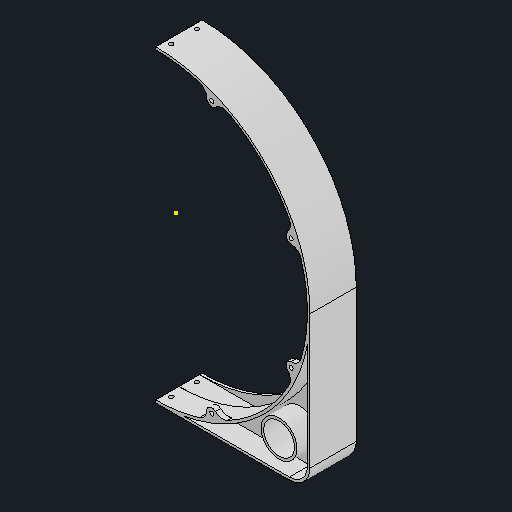
# Autodesk Inventor part: 3DPRINT,CABLE-SHROUD,OUTER
Saved by Autodesk Inventor 2026 (Build 300175000, 175)
## iProperties
Created: 2026-02-11
Part Number: 3DPRINT,CABLE-SHROUD,OUTER
Material: Generic
Document SubType Name: Modeling
Designer: littl
Density: 1 g/cm^3
Appearance: Default
Mass: 377.727 g
Surface Area: 2418.76 cm^2
Volume: 377.727 cm^3
Author: littl
Autodesk Inventor part; units mm, degrees
ref_plane "YZ Plane" through (0, 0, 0) normal (1, 0, 0) x (0, 1, 0)
ref_plane "XZ Plane" through (0, 0, 0) normal (0, 1, 0) x (-1, 0, 0)
ref_plane "XY Plane" through (0, 0, 0) normal (0, 0, 1) x (1, 0, 0)
sketch "Sketch1" plane through (0, 0, 0) normal (0, 0, 1) x (1, 0, 0)
  arc A0 (190.5, 0) -> (-190.5, 0) centre (0, 0) ccw
  circle A1 centre (0, 0) radius 187.325
  line L0 (-190.5, 0) -> (-190.5, -165.1)
  line L1 (-165.1, -190.5) -> (165.1, -190.5)
  line L2 (190.5, -165.1) -> (190.5, 0)
  arc A2 (-190.5, -165.1) -> (-165.1, -190.5) centre (-165.1, -165.1) ccw
  arc A3 (165.1, -190.5) -> (190.5, -165.1) centre (165.1, -165.1) ccw
  dimension "d0" = 381
  dimension "d1" = 3.175
  dimension "d2" = 25.4
  constraints: 7 tangent, 6 end point, 6 point on circle, 4 centre point, 2 coincident, 2 perpendicular, 1 equal radius, 1 vertical
  measures "d0" diameter of A0
  measures "d1" radial gap between concentric circles of A1 A0
  measures "d2" radius of A2
extrude "Extrusion1" add sketch "Sketch1" along normal blind 3.175
sketch "Sketch2" plane through (0, 0, 3.175) normal (0, 0, 1) x (1, 0, 0)
  line L0 (-190.5, 0) -> (-190.5, -165.1) projected
  arc A0 (-190.5, -165.1) -> (-165.1, -190.5) centre (-165.1, -165.1) ccw projected
  line L1 (-165.1, -190.5) -> (165.1, -190.5) projected
  arc A1 (165.1, -190.5) -> (190.5, -165.1) centre (165.1, -165.1) ccw projected
  line L2 (190.5, -165.1) -> (190.5, 0) projected
  arc A2 (190.5, 0) -> (-190.5, 0) centre (0, 0) ccw projected
  circle A3 centre (0, 0) radius 187.325 projected
  line L3 (-187.325, 0) -> (-187.325, -161.925)
  line L4 (187.325, 0) -> (187.325, -161.925)
  line L5 (161.925, -187.325) -> (-161.925, -187.325)
  circle A4 centre (0, 0) radius 187.325 projected
  arc A5 (-187.325, -161.925) -> (-161.925, -187.325) centre (-161.925, -161.925) ccw
  arc A6 (161.925, -187.325) -> (187.325, -161.925) centre (161.925, -161.925) ccw
  dimension "d5" = 25.4
  constraints: 7 tangent, 6 end point, 6 point on circle, 2 centre point, 2 perpendicular, 1 equal radius, 1 vertical
  measures "d5" radius of A5
extrude "Extrusion2" add sketch "Sketch2" along normal blind 12.7
mirror "Mirror1" about plane through (0, 0, 15.875) normal (0, 0, 1) of "Extrusion1", "Extrusion2"
sketch "Sketch3" plane through (0, 0, 31.75) normal (0, 0, 1) x (1, 0, 0)
  point P0 (0, 0)
sketch "Sketch4" plane through (0, 0, 31.75) normal (0, 0, -1) x (-1, 0, 0)
  line L0 (190.5, 0) -> (190.5, -165.1) projected
  arc A0 (190.5, 0) -> (-190.5, 0) centre (0, 0) ccw projected
  line L1 (-190.5, -165.1) -> (-190.5, 0) projected
  arc A1 (-190.5, -165.1) -> (-165.1, -190.5) centre (-165.1, -165.1) ccw projected
  line L2 (165.1, -190.5) -> (-165.1, -190.5) projected
  arc A2 (165.1, -190.5) -> (190.5, -165.1) centre (165.1, -165.1) ccw projected
  circle A3 centre (0, 0) radius 187.325 projected
  arc A4 (-187.325, -165.1) -> (-165.1, -187.325) centre (-165.1, -165.1) ccw
  line L3 (-187.325, -165.1) -> (-187.325, 0)
  arc A5 (187.325, 0) -> (-187.325, 0) centre (0, 0) ccw
  line L4 (187.325, 0) -> (187.325, -165.1)
  arc A6 (165.1, -187.325) -> (187.325, -165.1) centre (165.1, -165.1) ccw
  line L5 (165.1, -187.325) -> (-165.1, -187.325)
  circle A7 centre (0, 0) radius 190.5
  point P0 (-34.6352, -187.325)
  point P1 (-187.325, -34.6352)
  point P2 (34.6352, -187.325)
  point P3 (187.325, -34.6352)
  dimension "d8" = 3.175
  dimension "d9" = 3.175
  constraints: 6 end point, 6 point on circle, 4 centre point, 5 other
  measures "d8" distance between parallel lines of L2 L5
  measures "d9" radial gap between concentric circles of A3 A7
extrude "Extrusion3" add sketch "Sketch4" against normal blind 25.4504 contours A7 L4 A3 L3 A0 | L0 A2 L2 A7 L5 A6 L4 | A7 L3 A4 L5 L2 A1 L1 | A7 L5 A3 L4 | L3 A3 L5 A7 | A7 L5
sketch "Sketch5" plane through (161.925, -187.325, 28.575) normal (0, 0, -1) x (-1, 0, 0)
  circle A0 centre (9.525, 34.925) radius 19.05
  point P0 (161.925, 187.325)
  dimension "d12" = 38.1
  dimension "d13" = 152.4
  dimension "d14" = 152.4
  constraints: 1 centre point
  measures "d12" diameter of A0
  measures "d13" horizontal distance of point (161.925, 187.325) A0.centre
  measures "d14" horizontal distance of point (161.925, 187.325) A0.centre
extrude "Extrusion4" cut sketch "Sketch5" against normal through all
sketch "Sketch6" plane through (34.6352, -187.325, 31.75) normal (0, 0, 1) x (1, 0, 0)
  circle A0 centre (117.7648, 34.925) radius 19.05 projected
  circle A1 centre (117.7648, 34.925) radius 19.05
  circle A2 centre (117.7648, 34.925) radius 22.225
  point P0 (-34.6352, 187.325)
  dimension "d17" = 3.175
  constraints: 2 centre point, 2 coincident
  measures "d17" radial gap between concentric circles of A0 A2
extrude "Extrusion5" add sketch "Sketch6" along normal up to surface (25.4504 mm away)
sketch "Sketch7" plane through (0, 0, 0) normal (1, 0, 0) x (0, 1, 0)
  line L0 (-211.2628, -72.6551) -> (211.2628, -72.6551)
  line L1 (211.2628, -72.6551) -> (211.2628, 72.6551)
  line L2 (211.2628, 72.6551) -> (-211.2628, 72.6551)
  line L3 (-211.2628, 72.6551) -> (-211.2628, -72.6551)
  line L4 (-211.2628, -72.6551) -> (211.2628, 72.6551) construction
  line L5 (211.2628, -72.6551) -> (-211.2628, 72.6551) construction
  point P0 (0, 0)
  constraints: 12 end point, 2 midpoint, 2 parallel, 1 horizontal, 1 perpendicular
extrude "Extrusion6" cut sketch "Sketch7" against normal through all
sketch "Sketch8" plane through (165.1, -190.5, 0) normal (0, -1, 0) x (1, 0, 0)
  line L0 (-165.1, 0) -> (0, 0) projected
  line L1 (-165.1, 57.2004) -> (-165.1, 0) projected
  point P0 (-158.75, 12.7)
  point P1 (-158.75, 44.45)
  dimension "d22" = 12.7
  dimension "d23" = 31.75
  dimension "d24" = 6.35
  constraints: 1 vertical alignment
  measures "d22" distance from line of L0 point (-158.75, 12.7)
  measures "d23" distance of point (-158.75, 12.7) point (-158.75, 44.45)
  measures "d24" distance from line of L1 point (-158.75, 12.7)
hole "Hole1" at (6.35, -190.5, 44.45) at (6.35, -190.5, 12.7) direction (0, 1, 0) diameter 5.08 end through all
sketch "Sketch9" plane through (0, 0, 57.2004) normal (0, 0, 1) x (1, 0, 0)
  arc A0 (0, -187.325) -> (187.325, 0) centre (0, 0) ccw projected
  line L0 (69.2561, -167.1991) -> (0, 0) construction
  line L1 (-45.2243, 0) -> (271.3455, 0) projected
  line L2 (0, 0) -> (0, -221.1499)
  circle A1 centre (69.2561, -167.1991) radius 6.35
  arc A2 (73.7587, -162.7215) -> (66.8261, -161.3325) centre (69.2561, -167.1991) ccw
  arc A3 (66.8261, -161.3325) -> (62.9062, -167.2167) centre (69.2561, -167.1991) ccw
  arc A4 (73.7587, -162.7215) -> (88.7831, -164.9492) centre (82.7639, -153.7662) ccw
  arc A5 (53.8576, -179.4158) -> (62.9062, -167.2167) centre (50.2062, -167.252) ccw
  arc A6 (0, -187.325) -> (0, 187.325) centre (0, 0) ccw projected
  circle A7 centre (167.1991, -69.2561) radius 6.35
  arc A8 (164.9492, -88.7831) -> (162.7215, -73.7587) centre (153.7662, -82.7639) ccw
  arc A9 (167.2167, -62.9062) -> (179.4158, -53.8576) centre (167.252, -50.2062) ccw
  circle A10 centre (167.1991, 69.2561) radius 6.35
  arc A11 (179.4158, 53.8576) -> (167.2167, 62.9062) centre (167.252, 50.2062) ccw
  arc A12 (162.7215, 73.7587) -> (164.9492, 88.7831) centre (153.7662, 82.7639) ccw
  circle A13 centre (69.2561, 167.1991) radius 6.35
  arc A14 (88.7831, 164.9492) -> (73.7587, 162.7215) centre (82.7639, 153.7662) ccw
  arc A15 (62.9062, 167.2167) -> (53.8576, 179.4158) centre (50.2062, 167.252) ccw
  circle A16 centre (-69.2561, 167.1991) radius 6.35
  arc A17 (-53.8576, 179.4158) -> (-62.9062, 167.2167) centre (-50.2062, 167.252) ccw
  arc A18 (-73.7587, 162.7215) -> (-88.7831, 164.9492) centre (-82.7639, 153.7662) ccw
  circle A19 centre (-167.1991, 69.2561) radius 6.35
  arc A20 (-164.9492, 88.7831) -> (-162.7215, 73.7587) centre (-153.7662, 82.7639) ccw
  arc A21 (-167.2167, 62.9062) -> (-179.4158, 53.8576) centre (-167.252, 50.2062) ccw
  circle A22 centre (-167.1991, -69.2561) radius 6.35
  arc A23 (-179.4158, -53.8576) -> (-167.2167, -62.9062) centre (-167.252, -50.2062) ccw
  arc A24 (-162.7215, -73.7587) -> (-164.9492, -88.7831) centre (-153.7662, -82.7639) ccw
  circle A25 centre (-69.2561, -167.1991) radius 6.35
  arc A26 (-88.7831, -164.9492) -> (-73.7587, -162.7215) centre (-82.7639, -153.7662) ccw
  arc A27 (-62.9062, -167.2167) -> (-53.8576, -179.4158) centre (-50.2062, -167.252) ccw
  point P0 (161.3325, -66.8261)
  point P1 (161.3325, 66.8261)
  point P2 (66.8261, 161.3325)
  point P3 (-66.8261, 161.3325)
  point P4 (-161.3325, 66.8261)
  point P5 (-161.3325, -66.8261)
  point P6 (-66.8261, -161.3325)
  point P7 (179.4158, -53.8576)
  dimension "d32" = 180.975
  dimension "d38" = 12.7
  dimension "d39" = 67.5
  dimension "d40" = 12.7
  dimension "d43" = 360
  constraints: 62 point on circle, 26 centre point, 6 tangent, 4 end point, 3 coincident, 3 equal radius, 1 point on line, 1 vertical, 89 other
  measures "d32" distance of point (0, 0) L0.start
  measures "d38" diameter of A1
  measures "d39" angle of L1 L0
  measures "d40" radius of A4
extrude "Extrusion7" add sketch "Sketch9" against normal blind 6.35 contours A14 A13 A6 | A11 A10 A6 | A5 A1 A0 | A1 A4 A0 | A1 | A0 A7 A9 | A8 A7 A0 | A7 | A10 A12 A6 | A10 | A13 A15 A6 | A13
hole "Hole2" at (69.2561, -167.1991, 57.2004) at (167.1991, 69.2561, 57.2004) at (69.2561, 167.1991, 57.2004) at (167.1991, -69.2561, 57.2004) direction (0, 0, -1) diameter 5.1054 end through all clearance for "Flat Head Machine Screw (82)" size "#10" standard "Ansi Unified Screw Threads"
body "Solid1"
